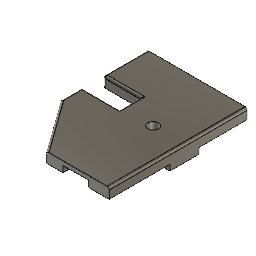
Panel-Cover V1 (Autodesk Fusion 360 design; units mm, degrees)
Autodesk Fusion 360 part; units mm, degrees
box "Grundkörper Quader1" add length 66 width 48 height 5 placed x (0, 1, 0) y (-1, 0, 0) z (0, 0, 1) at (48, 0, 0) makes body 1
box "Grundkörper Quader2" add length 21 width 6 height 1 placed x (0, -1, 0) y (1, 0, 0) z (0, 0, 1) at (-6, 66, 0) bodies 1
box "Grundkörper Quader3" cut length 10 width 18 height -5 placed x (0, 1, 0) y (-1, 0, 0) z (0, 0, 1) at (18, 35, 5) bodies 1
delete_face "Fläche löschen1" 1 faces at (-2, 59, 1) on bodies 1
sketch "Skizze6" plane through (0, 0, 5) normal (0, 0, 1) x (-1, 0, 0)
  line L0 (0, -45) -> (-18, -45)
  line L1 (-18, -45) -> (-18, -35)
  line L2 (-18, -35) -> (0, -35)
  line L3 (0, -35) -> (0, 0)
  line L4 (0, 0) -> (-48, 0)
  line L5 (-48, 0) -> (-48, -66)
  line L6 (-48, -66) -> (0, -66)
  line L7 (0, -66) -> (0, -45)
  line L8 (0, -25) -> (-18, 0)
  constraint coincident L3 L8.start
  constraint coincident L4 L8.end
split "Teilen1" by curves path "Skizze6" along L8 bodies 1 makes body 2 at (6, 8.3333, 5)
split_face "Fläche trennen1" 1 faces at (39.2801, 37, 5) by plane through (48, 0, 5) normal (0, 0, 1) on bodies 1
combine "Kombinieren1" operation cut target body 1 tool bodies 2
box "Grundkörper Quader7" add length 14 width 25 height 2.8 placed x (0, -1, 0) y (-1, 0, 0) z (0, 0, -1) at (48, 43.012, 0) separate body makes body 3
sketch "Skizze9" plane through (0, 0, 0) normal (0, 0, -1) x (1, 0, 0)
  line L0 (18, 0) -> (0, -25)
  line L1 (0, -25) -> (0, -35)
  line L2 (0, -35) -> (18, -35)
  line L3 (18, -35) -> (18, -45)
  line L4 (18, -45) -> (0, -45)
  line L5 (0, -45) -> (0, -66)
  line L6 (0, -66) -> (48, -66)
  line L7 (48, -66) -> (48, 0)
  line L8 (48, 0) -> (18, 0)
  line L9 (4.0465, -35) -> (26, -5)
  line L10 (26, -5) -> (26, 0)
  line L11 (38, 0) -> (38, -5)
  line L12 (38, -5) -> (18, -35)
  constraint coincident L2 L9.start
  constraint coincident L8 L10.end
  constraint perpendicular L8 L10
  constraint coincident L8 L11.start
  constraint perpendicular L8 L11
  constraint coincident L2.end L3.start
extrude "Extrusion1" cut sketch "Skizze9" against normal blind 3 contours L2 L8 L9 L10 L11 L12 bodies 1
combine "Kombinieren2" operation add target body 1 tool bodies 3
hole "Bohrung1" at (33, 36.012, -2.8) direction (0, 0, 1) diameter 5 depth 10 tip angle 180 bodies 1
fillet "Abrundung1" radius 1 11 edges at (0, 55.5, 5) (0, 45, 2.5) (9, 45, 5) (18, 40, 5) (9, 12.5, 5) (0, 30, 5) (9, 35, 5) (18, 35, 1.5) (11.0232, 35, 3) (4.0465, 35, 1.5) (48, 33, 5) on bodies 1
fillet "Abrundung2" radius 3 1 edges at (26, 5, 1.5) on bodies 1
fillet "Abrundung3" radius 3 1 edges at (38, 5, 1.5) on bodies 1
fillet "Abrundung4" radius 4 2 edges at (23, 29.012, -1.4) (23, 43.012, -1.4) on bodies 1
